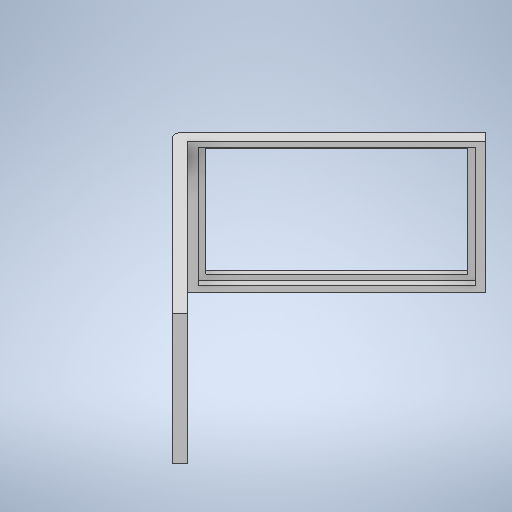
# Autodesk Inventor part: SolarPannelMounting
Saved by Autodesk Inventor 2025.2 (Build 292293000, 293)
## iProperties
Created: 2025-07-25
Part Number: SolarPannelMounting
Material: Generic
Document SubType Name: Modeling
Designer: arbaz
Density: 1 g/cm^3
Appearance: Default
Author: arbaz
Autodesk Inventor part; units mm, degrees
ref_plane "YZ Plane" through (0, 0, 0) normal (1, 0, 0) x (0, 1, 0)
ref_plane "XZ Plane" through (0, 0, 0) normal (0, 1, 0) x (-1, 0, 0)
ref_plane "XY Plane" through (0, 0, 0) normal (0, 0, 1) x (1, 0, 0)
sketch "Sketch4" plane through (0, 0, 0) normal (0, 1, 0) x (-1, 0, 0)
  line L0 (0, 0) -> (-71.842, 71.842)
  line L1 (0, 0) -> (101.6, 0) construction
  line L2 (0, 0) -> (-71.842, -71.842)
  line L3 (0, 0) -> (101.6, 0) construction
  line L4 (-71.842, 71.842) -> (-75.3776, 68.3065)
  line L5 (-75.3776, 68.3065) -> (-7.0711, 0)
  line L6 (-7.0711, 0) -> (-75.3776, -68.3065)
  line L7 (-75.3776, -68.3065) -> (-71.842, -71.842)
  dimension "d20" = 101.6
  dimension "d21" = 135
  dimension "d22" = 101.6
  dimension "d23" = 135
  dimension "d24" = 5
  constraints: 16 end point, 3 perpendicular, 2 equal length, 2 horizontal
  measures "d20" distance of L0.start L0.end
  measures "d21" angle of L1 L0
  measures "d22" distance of L0.start L2.end
  measures "d23" angle of L2 L3
  measures "d24" distance of L0.end L4.end
extrude "Extrusion3" add sketch "Sketch4" along normal blind 60
sketch "Sketch5" plane through (7.0711, 0, 0) normal (0.7071, 0, -0.7071) x (-0.7071, 0, -0.7071)
  line L0 (-96.6, 0) -> (0, 0) projected
  line L1 (0, 0) -> (0, 60) projected
  line L2 (-96.6, 60) -> (0, 60) projected
  line L3 (-96.6, 0) -> (-96.6, 60) projected
  line L4 (-96.6, 0) -> (0, 0) projected
  line L5 (-96.6, 60) -> (0, 0)
  line L6 (0, 0) -> (-96.6, 0)
  line L7 (0, 60) -> (5, 60) projected
  line L8 (-96.6, 0) -> (0, 60)
  line L9 (-93.3, 2.5) -> (-3.3, 2.5)
  line L10 (-3.3, 2.5) -> (-3.3, 57.5)
  line L11 (-3.3, 57.5) -> (-93.3, 57.5)
  line L12 (-93.3, 57.5) -> (-93.3, 2.5)
  line L13 (-93.3, 2.5) -> (-3.3, 57.5) construction
  line L14 (-3.3, 2.5) -> (-93.3, 57.5) construction
  point P0 (5, 0)
  point P1 (-48.3, 30)
  dimension "d27" = 90
  dimension "d28" = 55
  constraints: 18 end point, 3 equal length, 3 midpoint, 1 horizontal, 1 perpendicular
  measures "d27" distance of L11.end L10.end
  measures "d28" distance of L10.end L9.end
extrude "Extrusion4" cut sketch "Sketch5" against normal blind 3 contours L9 L12 L11 L5 L8 | L8 L5 L9 | L5 L8 L11 L10 L9 | L11 L8 L5
sketch "Sketch6" plane through (4.9497, 0, 2.1213) normal (0.7071, 0, -0.7071) x (-0.7071, 0, -0.7071)
  line L0 (-93.3, 2.5) -> (-93.3, 57.5) projected
  line L1 (-3.3, 2.5) -> (-93.3, 2.5) projected
  line L2 (-3.3, 57.5) -> (-3.3, 2.5) projected
  line L3 (-93.3, 57.5) -> (-3.3, 57.5) projected
  line L4 (-90.8, 5) -> (-5.8, 5)
  line L5 (-5.8, 5) -> (-5.8, 55)
  line L6 (-5.8, 55) -> (-90.8, 55)
  line L7 (-90.8, 55) -> (-90.8, 5)
  line L8 (-90.8, 5) -> (-5.8, 55) construction
  line L9 (-5.8, 5) -> (-90.8, 55) construction
  point P0 (5, 0)
  point P1 (-48.3, 30)
  dimension "d31" = 85
  dimension "d32" = 50
  constraints: 12 end point, 2 midpoint, 2 parallel, 1 horizontal, 1 perpendicular
  measures "d31" distance of L6.end L5.end
  measures "d32" distance of L5.end L4.end
extrude "Extrusion5" cut sketch "Sketch6" against normal blind 3 contours L7 L6 L5 L4
sketch "Sketch7" plane through (75.3776, 0, -68.3065) normal (0.7071, 0, 0.7071) x (0.7071, 0, -0.7071)
  line L0 (-96.6, 0) -> (0, 0) projected
  line L1 (0, 0) -> (0, 60) projected
  line L2 (-96.6, 60) -> (0, 60) projected
  line L3 (-96.6, 0) -> (-96.6, 60) projected
  line L4 (-96.6, 0) -> (0, 60)
  line L5 (-96.6, 60) -> (0, 0)
  line L6 (-93.3, 2.5) -> (-3.3, 2.5)
  line L7 (-3.3, 2.5) -> (-3.3, 57.5)
  line L8 (-3.3, 57.5) -> (-93.3, 57.5)
  line L9 (-93.3, 57.5) -> (-93.3, 2.5)
  line L10 (-93.3, 2.5) -> (-3.3, 57.5) construction
  line L11 (-3.3, 2.5) -> (-93.3, 57.5) construction
  point P0 (-101.6, 0)
  point P1 (-48.3, 30)
  dimension "d35" = 90
  dimension "d36" = 55
  constraints: 16 end point, 3 midpoint, 2 parallel, 1 horizontal, 1 perpendicular
  measures "d35" distance of L8.end L7.end
  measures "d36" distance of L7.end L6.end
extrude "Extrusion6" cut sketch "Sketch7" against normal blind 3 contours L6 L9 L8 L5 L4 | L4 L5 L6 | L5 L4 L8 L7 L6 | L8 L4 L5
sketch "Sketch8" plane through (73.2563, 0, -70.4278) normal (0.7071, 0, 0.7071) x (0.7071, 0, -0.7071)
  line L0 (-93.3, 2.5) -> (-93.3, 57.5) projected
  line L1 (-3.3, 2.5) -> (-93.3, 2.5) projected
  line L2 (-3.3, 57.5) -> (-3.3, 2.5) projected
  line L3 (-93.3, 57.5) -> (-3.3, 57.5) projected
  line L4 (-90.8, 5) -> (-5.8, 5)
  line L5 (-5.8, 5) -> (-5.8, 55)
  line L6 (-5.8, 55) -> (-90.8, 55)
  line L7 (-90.8, 55) -> (-90.8, 5)
  line L8 (-90.8, 5) -> (-5.8, 55) construction
  line L9 (-5.8, 5) -> (-90.8, 55) construction
  point P0 (-101.6, 0)
  point P1 (-48.3, 30)
  dimension "d39" = 85
  dimension "d40" = 50
  constraints: 12 end point, 2 midpoint, 2 parallel, 1 horizontal, 1 perpendicular
  measures "d39" distance of L6.end L5.end
  measures "d40" distance of L5.end L4.end
extrude "Extrusion7" cut sketch "Sketch8" against normal blind 3 contours L7 L6 L5 L4
fillet "Fillet1" radius 3.175 1 edges at (0, 30, 0)
body "Solid2"
